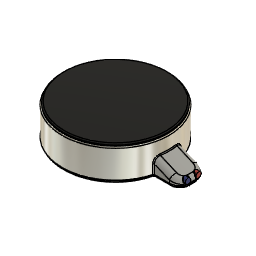
Vibrations (Autodesk Fusion 360 design; units mm, degrees)
Autodesk Fusion 360 part; units mm, degrees
sketch "Sketch1" plane through (0, 0, 0) normal (0, 0, 1) x (1, 0, 0)
  circle A0 centre (0, 0) radius 5
  dimension "d17" = 10
  constraint coincident A0.centre origin
  measures "d17" diameter of A0
extrude "Extrude5" add sketch "Sketch1" along normal blind 3.2
sketch "Sketch2" plane through (0, 0, 0) normal (0, 0, -1) x (1, 0, 0)
  circle A0 centre (0, 0) radius 5
  circle A1 centre (0, 0) radius 4.9
  dimension "d20" = -0.1
extrude "Extrude6" cut sketch "Sketch2" against normal blind 0.2
fillet "Fillet1" radius 0.1 2 edges at (-4.6616, -1.8081, 0.2) (-4.5684, 1.7719, 0)
sketch "Sketch3" plane through (0, 0, 3.2) normal (0, 0, 1) x (-1, 0, 0)
  circle A0 centre (0, 0) radius 5
  circle A1 centre (0, 0) radius 4.9
  dimension "d25" = -0.1
extrude "Extrude7" cut sketch "Sketch3" against normal blind 0.2
fillet "Fillet2" radius 0.1 2 edges at (4.5684, 1.7719, 3.2) (-4.6616, 1.8081, 3)
sketch "Sketch4" plane through (0, 0, 0) normal (0, 0, -1) x (1, 0, 0)
  circle A0 centre (0, 0) radius 4.8
  line L0 (0, 0) -> (4.8, 0)
  line L1 (4.8, 0) -> (4.8, -1.25)
  line L2 (4.8, -1.25) -> (4.8, 0)
  line L3 (4.8, 0) -> (4.8, 1.25)
  line L4 (4.8, 1.25) -> (7.3, 1.25)
  line L5 (7.3, 1.25) -> (7.3, -1.25)
  line L6 (7.3, -1.25) -> (4.8, -1.25)
  line L7 (4.8, -1.25) -> (4.8, 1.25)
  line L8 (4.8, 1.25) -> (4.6344, 1.25)
  line L9 (4.8, -1.25) -> (4.6344, -1.25)
  dimension "d30" = 1.25
  dimension "d31" = 1.25
  dimension "d32" = 2.5
  dimension "d33" = 2.5
  constraint coincident A0.centre L0.start
  constraint coincident A0 L0.end
  constraint horizontal L0
  constraint perpendicular L0 L1
  constraint perpendicular L0 L3
  constraint horizontal L4
  constraint vertical L5
  constraint horizontal L6
  constraint vertical L7
  constraint coincident A0 L8.end
  constraint perpendicular L3 L8
  constraint coincident A0 L9.end
  constraint perpendicular L7 L9
  measures "d30" distance of L0.end L1.end
  measures "d31" distance of L0.end L3.end
  measures "d32" distance of L3.end L4.end
  measures "d33" distance of L3.end L1.end
extrude "Extrude8" add sketch "Sketch4" against normal blind 0.7 contours A0 L1 L2 L7 L9 | L1 L2 L3 L4 L5 L6 L7 | A0 L3 L7 L8
fillet "Fillet3" radius 1 2 edges at (7.3, -1.25, 0.35) (7.3, 1.25, 0.35)
chamfer "Chamfer1" distance 1 distance2 2.3 1 edges at (5, 0, 0.7) measured on face at (-5, 0, 2.0333)
fillet "Fillet4" radius 0.5 7 edges at (5.4879, -1.25, 1.4268) (6.941, -1.0175, 0.8238) (5.4879, 1.25, 1.4268) (6.941, 1.0175, 0.8238) (7.2973, 0.1983, 0.7) (7.2973, -0.3234, 0.7) (7.3, -0.125, 0.7)
sketch "Sketch5" plane through (0, 0, 0) normal (0, 0, -1) x (1, 0, 0)
  arc A0 (6.3, -1.25) -> (7.3, -0.25) centre (6.3, -0.25) ccw
  line L0 (7.3, -0.25) -> (7.3, 0.25)
  arc A1 (7.3, 0.25) -> (6.3, 1.25) centre (6.3, 0.25) ccw
  line L1 (6.3, 1.25) -> (4.6344, 1.25)
  arc A2 (4.6344, 1.25) -> (4.6344, -1.25) centre (0, 0) ccw
  line L2 (4.6344, -1.25) -> (6.3, -1.25)
  line L3 (4.5571, -1.15) -> (6.3, -1.15)
  arc A3 (6.3, -1.15) -> (7.2, -0.25) centre (6.3, -0.25) ccw
  line L4 (7.2, -0.25) -> (7.2, 0.25)
  arc A4 (7.2, 0.25) -> (6.3, 1.15) centre (6.3, 0.25) ccw
  line L5 (6.3, 1.15) -> (4.5571, 1.15)
  arc A5 (4.5571, 1.15) -> (4.5571, -1.15) centre (0, 0) ccw
  circle A6 centre (0, 0) radius 4.8
  line L6 (4.7379, -1.25) -> (4.6344, -1.25)
  arc A7 (4.6344, 1.25) -> (4.6344, -1.25) centre (0, 0) ccw
  line L7 (4.6344, 1.25) -> (4.7379, 1.25)
  arc A8 (4.7379, 1.25) -> (4.7379, -1.25) centre (0, 0) ccw
  circle A9 centre (0, 0) radius 4.9
  dimension "d42" = -0.1
  constraint concentric A2 A6
  constraint coincident A2.end A6
  constraint concentric A6 A9
  constraint coincident L6.start A9
extrude "Extrude9" cut sketch "Sketch5" against normal blind 0.2 contours A0 L0 A1 L1 L2 L3 A3 L4 A4 L5 A9
fillet "Fillet5" radius 0.1 7 edges at (4.7508, 1.2001, 0) (5.5316, 1.15, 0) (6.9364, 0.8864, 0) (7.2, 0, 0) (6.9364, -0.8864, 0) (5.5316, -1.15, 0) (4.7508, -1.2001, 0)
fillet "Fillet6" radius 0.1 4 edges at (4.7367, 1.1166, 0.0254) (4.7631, 1.15, 0.15) (4.7367, -1.1166, 0.0254) (4.7631, -1.15, 0.15)
fillet "Fillet7" radius 0.1 5 edges at (5.5189, -1.25, 0.2) (7.0071, -0.9571, 0.2) (7.3, 0, 0.2) (7.0071, 0.9571, 0.2) (5.5189, 1.25, 0.2)
fillet "Fillet8" radius 0.1 7 edges at (4.8218, -1.225, 0.2338) (4.8412, -1.25, 0.7494) (4.873, -1.1196, 1.5516) (5, 0, 1.7) (4.8731, 1.1194, 1.5518) (4.8412, 1.25, 0.7494) (4.8218, 1.225, 0.2338)
sketch "Sketch6" plane through (7.3, 0, 0) normal (1, 0, 0) x (0, 1, 0)
  line L0 (-0.25, 0.3) -> (0.25, 0.3)
  line L1 (0.25, 0.3) -> (0.25, 0.3702)
  spline S0 degree 3 poles (-0.25, 0.3702) (-0.0834, 0.3728) (0.0833, 0.3728) (0.25, 0.3702) knots -0.200397 -0.200397 -0.200397 -0.200397 -0.150412 -0.150412 -0.150412 -0.150412
  line L2 (-0.25, 0.3702) -> (-0.25, 0.3)
  circle A0 centre (-0.5, 0.6) radius 0.25
  dimension "d53" = 0.5
  dimension "d54" = 0.5
  dimension "d55" = 0.6
  measures "d53" diameter of A0
  measures "d54" horizontal distance of origin A0.centre
  measures "d55" vertical distance of origin A0.centre
extrude "Extrude10" add sketch "Sketch6" against normal blind 0.55 contours A0
fillet "Fillet9" radius 0.05 6 edges at (7.2414, -0.25, 0.605) (7.2924, -0.3007, 0.449) (7.2649, -0.5126, 0.3503) (7.0719, -0.7355, 0.684) (6.9483, -0.4576, 0.8464) (7.0844, -0.3255, 0.7791)
mirror "Mirror1" about plane through (0, 0, 0) normal (0, 1, 0) of "Extrude10", "Fillet9"
named bodies: "Vibrations"
